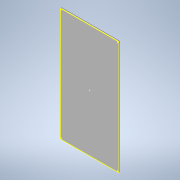
# Autodesk Inventor part: oled_mask
Saved by Autodesk Inventor 2021 (Build 250183000, 183)
## iProperties
Created: 2021-01-06
Part Number: oled_mask
Material: Generic
Document SubType Name: Modeling
Designer: lgnds
Density: 1 g/cm^3
Appearance: Default
Author: lgnds
Autodesk Inventor part; units mm, degrees
ref_plane "YZ Plane" through (0, 0, 0) normal (1, 0, 0) x (0, 1, 0)
ref_plane "XZ Plane" through (0, 0, 0) normal (0, 1, 0) x (-1, 0, 0)
ref_plane "XY Plane" through (0, 0, 0) normal (0, 0, 1) x (1, 0, 0)
sketch "Sketch1" plane through (0, 0, 0) normal (0, 0, 1) x (1, 0, 0)
  line L0 (-14.75, -28.5) -> (14.75, -28.5)
  line L1 (14.75, -28.5) -> (14.75, 28.5)
  line L2 (14.75, 28.5) -> (-14.75, 28.5)
  line L3 (-14.75, 28.5) -> (-14.75, -28.5)
  line L4 (-14.75, -28.5) -> (14.75, 28.5) construction
  line L5 (14.75, -28.5) -> (-14.75, 28.5) construction
  point P0 (0, 0)
  dimension "d0" = 29.5
  dimension "d1" = 57
  constraints: 12 end point, 2 midpoint, 2 parallel, 1 horizontal, 1 perpendicular
  measures "d0" distance between parallel lines of L1 L3
  measures "d1" distance between parallel lines of L0 L2
extrude "Extrusion1" add sketch "Sketch1" along normal blind 0.5
fillet "Fillet1" radius 0.5 4 edges at (-14.75, -28.5, 0.25) (14.75, -28.5, 0.25) (14.75, 28.5, 0.25) (-14.75, 28.5, 0.25)
sketch "Sketch3" plane through (0, 0, 0.5) normal (0, 0, 1) x (1, 0, 0)
  arc A0 (-14.25, 28.5) -> (-14.75, 28) centre (-14.25, 28) ccw projected
  line L0 (-14.75, 28) -> (-14.75, -28) projected
  arc A1 (-14.75, -28) -> (-14.25, -28.5) centre (-14.25, -28) ccw projected
  line L1 (-14.25, -28.5) -> (14.25, -28.5) projected
  arc A2 (14.25, -28.5) -> (14.75, -28) centre (14.25, -28) ccw projected
  line L2 (14.75, -28) -> (14.75, 28) projected
  arc A3 (14.75, 28) -> (14.25, 28.5) centre (14.25, 28) ccw projected
  line L3 (14.25, 28.5) -> (-14.25, 28.5) projected
  point P0 (0, 0)
body "Solid1"
